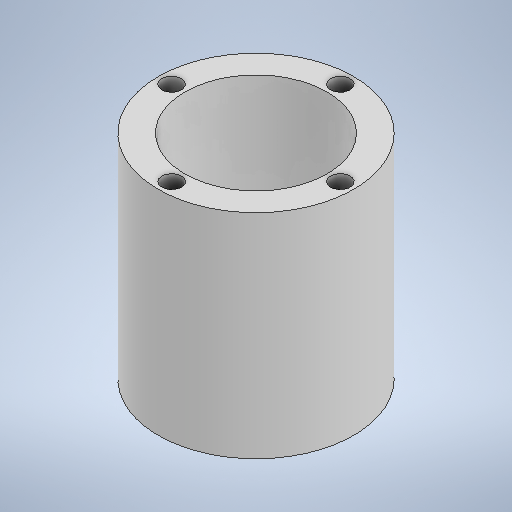
# Autodesk Inventor part: cilindro
Saved by Autodesk Inventor 2025.2 (Build 292293000, 293)
## iProperties
Created: 2026-09-20
Part Number: cilindro
Material: Generic
Document SubType Name: Sheet Metal
Designer: dguar
Density: 1 g/cm^3
Sheet Metal Rule: Default_mm
Appearance: Default
Author: dguar
Autodesk Inventor part; units mm, degrees
ref_plane "YZ Plane" through (0, 0, 0) normal (1, 0, 0) x (0, 1, 0)
ref_plane "XZ Plane" through (0, 0, 0) normal (0, 1, 0) x (-1, 0, 0)
ref_plane "XY Plane" through (0, 0, 0) normal (0, 0, 1) x (1, 0, 0)
sketch "Sketch1" plane through (0, 0, 0) normal (0, 1, 0) x (-1, 0, 0)
  circle A0 centre (0, 0) radius 40
  circle A1 centre (0, 0) radius 55
  circle A2 centre (47.5, 0) radius 5.5
  circle A3 centre (0, -47.5) radius 5.5
  circle A4 centre (0, 47.5) radius 5.5
  circle A5 centre (-47.5, 0) radius 5.5
  dimension "d0" = 80
  dimension "d10" = 11
  dimension "d11" = 11
  dimension "d12" = 11
  dimension "d13" = 11
  constraints: 6 centre point, 2 coincident
  measures "d0" diameter of A0
  measures "d10" diameter of A2
  measures "d11" diameter of A3
  measures "d12" diameter of A4
  measures "d13" diameter of A5
extrude "Extrusion1" add sketch "Sketch1" along normal blind 120
equation "\"BendRadius\" = Thickness"
equation "\"BendReliefWidth\" = Thickness"
equation "\"BendReliefDepth\" = 0.5 * Thickness"
equation "\"CornerReliefSize\" = 4 * Thickness"
equation "\"MinimumRemnant\" = 2 * Thickness"
equation "\"TransitionRadius\" = BendRadius"
equation "\"JacobiRadiusSize\" = BendRadius"
equation "\"GapSize\" = Thickness"
equation "\"Thickness\" = 0.5"
body "Solid1"
